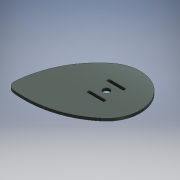
# Autodesk Inventor part: leva00
Saved by Autodesk Inventor 2016 (Build 200138000, 138)
## iProperties
Created: 2016-09-20
Part Number: leva00
Material: Madera (abedul)
Document SubType Name: Modeling
Designer: i95sa
Density: 0.55 g/cm^3
Appearance: Gris plomo - Pulido
Author: i95sa
Autodesk Inventor part; units mm, degrees
ref_plane "YZ Plane" through (0, 0, 0) normal (1, 0, 0) x (0, 1, 0)
ref_plane "XZ Plane" through (0, 0, 0) normal (0, 1, 0) x (-1, 0, 0)
ref_plane "XY Plane" through (0, 0, 0) normal (0, 0, 1) x (1, 0, 0)
sketch "Boceto1" plane through (0, 0, 0) normal (0, 0, 1) x (1, 0, 0)
  arc A0 (38.5141, 31.8616) -> (-38.5141, -31.8616) centre (0, 0) ccw
  arc A1 (-59.2702, -49.0326) -> (-77.0459, -63.7379) centre (-68.158, -56.3852) ccw
  line L0 (-79.6192, -65.8667) -> (-86.9719, -56.9788)
  line L1 (-31.4032, 38.8888) -> (-43.6576, 53.7019)
  line L2 (-43.6576, 53.7019) -> (-86.9719, -56.9788)
  line L3 (-86.9719, -56.9788) -> (-70.157, -14.0119)
  arc A2 (-31.4032, 38.8888) -> (-70.157, -14.0119) centre (48.9563, -60.6261) ccw
  arc A3 (-70.157, -14.0119) -> (-79.6586, -55.4943) centre (64.3488, -66.6499) ccw
  line L4 (2.9626, 2.4509) -> (38.5141, 31.8616)
  line L5 (-2.9626, -2.4509) -> (-79.6192, -65.8667)
  arc A4 (-38.5141, -31.8616) -> (38.5141, 31.8616) centre (0, 0) ccw
  arc A5 (-77.0459, -63.7379) -> (-59.2702, -49.0326) centre (-68.158, -56.3852) ccw
  line L6 (-79.6192, -65.8667) -> (-72.2665, -74.7546)
  line L7 (32.3156, -38.134) -> (44.5701, -52.9471)
  line L8 (44.5701, -52.9471) -> (-72.2665, -74.7546)
  line L9 (-72.2665, -74.7546) -> (-26.9098, -66.2888)
  arc A6 (-26.9098, -66.2888) -> (32.3156, -38.134) centre (-50.3788, 59.4493) ccw
  arc A7 (-69.4379, -67.849) -> (-26.9098, -66.2888) centre (-53.4116, 75.698) ccw
  dimension "d0" = 99.97
  dimension "d6" = 23.07
  dimension "d7" = 11.535
  dimension "d8" = 19.225
  dimension "d9" = 46.14
  constraints: 20 end point, 20 point on circle, 8 centre point, 6 symmetric about line, 5 point on line, 4 tangent, 1 collinear, 4 other
  measures "d0" diameter of A0
  measures "d6" diameter of A1
  measures "d7" distance of L0.start L0.end
  measures "d8" distance of L1.start L1.end
  measures "d9" distance of L0.end L3.end
extrude "Extrusión2" add sketch "Boceto1" along normal blind 4 contours A4 A0 | A0 L5 A1 A3 A2 | A6 A7 A5 L5 A4 | L5 A1 | A5 L5
sketch "Boceto2" plane through (0, 0, 4) normal (0, 0, 1) x (1, 0, 0)
  line L0 (0, 0) -> (0, 12.5)
  line L1 (0, 12.5) -> (-12.5, 12.5)
  line L2 (-12.5, 12.5) -> (-12.5, 16.7)
  line L3 (-12.5, 16.7) -> (12.5, 16.7)
  line L4 (12.5, 16.7) -> (12.5, 12.5)
  line L5 (12.5, 12.5) -> (0, 12.5)
  line L6 (0, 0) -> (12.5, 0)
  line L7 (0, 0) -> (0, -12.5)
  line L8 (0, -12.5) -> (-12.5, -12.5)
  line L9 (-12.5, -12.5) -> (-12.5, -16.7)
  line L10 (-12.5, -16.7) -> (12.5, -16.7)
  line L11 (12.5, -16.7) -> (12.5, -12.5)
  line L12 (12.5, -12.5) -> (0, -12.5)
  circle A0 centre (0, 0) radius 5
  dimension "d24" = 12.5
  dimension "d25" = 12.5
  dimension "d26" = 4.2
  dimension "d27" = 25
  dimension "d28" = 10
  constraints: 26 end point, 5 perpendicular, 5 symmetric about line, 3 point on line, 1 centre point, 1 coincident, 1 parallel, 1 vertical
  measures "d24" distance of L0.start L0.end
  measures "d25" distance of L0.end L1.end
  measures "d26" distance of L1.end L2.end
  measures "d27" distance of L2.end L3.end
  measures "d28" diameter of A0
extrude "Extrusión3" cut sketch "Boceto2" against normal blind 4
